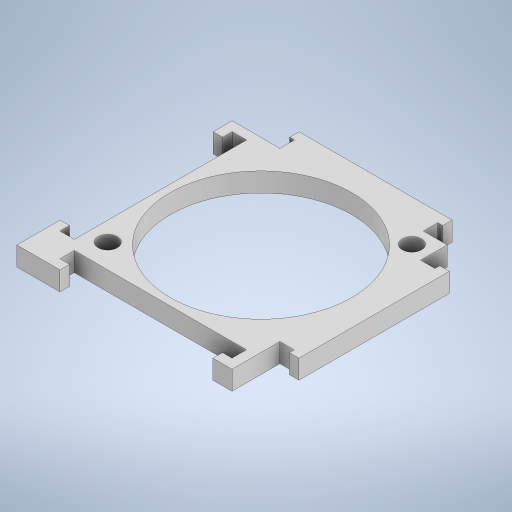
# Autodesk Inventor part: Maschio-femmina
Saved by Autodesk Inventor 2024 (Build 280153000, 153)
## iProperties
Created: 2024-01-14
Part Number: Maschio-femmina
Material: Generico
Document SubType Name: Modeling
Designer: Leonardo
Density: 1 g/cm^3
Appearance: Default
Author: Leonardo
Autodesk Inventor part; units mm, degrees
ref_plane "YZ Plane" through (0, 0, 0) normal (1, 0, 0) x (0, 1, 0)
ref_plane "XZ Plane" through (0, 0, 0) normal (0, 1, 0) x (-1, 0, 0)
ref_plane "XY Plane" through (0, 0, 0) normal (0, 0, 1) x (1, 0, 0)
sketch "Schizzo1" plane through (0, 0, 0) normal (0, 1, 0) x (-1, 0, 0)
  line L0 (10.0009, -10.0148) -> (9.0009, -10.0148)
  line L1 (-10, 9) -> (-10, 10)
  line L2 (11.5009, -9.0148) -> (10.0009, -9.0148)
  line L3 (10.0009, 8.9852) -> (10.0009, -9.0148)
  line L4 (-10, 12) -> (-10, 10)
  line L5 (9, 10) -> (-9, 10)
  line L6 (-10, -10.0148) -> (-9, -10.0148)
  line L7 (9.0009, -10.0148) -> (8.0009, -10.0148)
  line L8 (-9, -10.0148) -> (-8, -10.0148)
  line L9 (-10, 9) -> (-10, 8)
  line L10 (-10, -10.0148) -> (-10, -7.7324)
  circle A0 centre (-0.2724, -0.2591) radius 9.5
  line L11 (11.5009, -9.0148) -> (11.5009, -8.0148)
  line L12 (11.5009, -8.0148) -> (12.5009, -8.0148)
  line L13 (12.5009, -8.0148) -> (12.5009, -10.0148)
  line L14 (12.5009, -10.0148) -> (10.0009, -10.0148)
  line L15 (10.0009, 8.9852) -> (11.5009, 8.9852)
  line L16 (11.5009, 8.9852) -> (11.5009, 7.9852)
  line L17 (11.5009, 7.9852) -> (12.5009, 7.9852)
  line L18 (12.5009, 7.9852) -> (12.5009, 9.9852)
  line L19 (9, 10) -> (9, 11.5)
  line L20 (9, 11.5) -> (8, 11.5)
  line L21 (8, 11.5) -> (8, 12.5)
  line L22 (8, 12.5) -> (10, 12.5)
  line L23 (12.5009, 9.9852) -> (12.5009, 12.5)
  line L24 (12.5009, 12.5) -> (10, 12.5)
  line L25 (-9, 10) -> (-9, 11.5)
  line L26 (-9, 11.5) -> (-8, 11.5)
  line L27 (-8, 11.5) -> (-8, 12.5)
  line L28 (-8, 12.5) -> (-10, 12.5)
  line L29 (-10, 12.5) -> (-10, 12)
  line L30 (-10, -7.7324) -> (-10, -7.2324)
  line L31 (-10, 8) -> (-10, 7.5)
  line L32 (-10, 7.5) -> (-11, 7.5)
  line L33 (8.0009, -10.0148) -> (7.5009, -10.0148)
  line L34 (7.5009, -10.0148) -> (7.5009, -11.0148)
  line L35 (-8, -10.0148) -> (-7.5, -10.0148)
  line L36 (-7.5, -10.0148) -> (-7.5, -11.0148)
  line L37 (-10, -7.2324) -> (-11.5, -7.2324)
  line L38 (-11.5, -7.2324) -> (-11.5, -7.7324)
  line L39 (-11.5, -7.7324) -> (-12.5, -7.7324)
  line L40 (-11, 7.5) -> (-11.5, 7.5)
  line L41 (-11.5, 7.5) -> (-11.5, 8)
  line L42 (-11.5, 8) -> (-12.5, 8)
  line L43 (-12.5, -7.7324) -> (-12.5, 8)
  line L44 (-7.5, -11.0148) -> (-7.5, -11.5148)
  line L45 (-7.5, -11.5148) -> (-8, -11.5148)
  line L46 (-8, -11.5148) -> (-8, -12.5148)
  line L47 (7.5009, -11.0148) -> (7.5009, -11.5148)
  line L48 (7.5009, -11.5148) -> (8.0009, -11.5148)
  line L49 (8.0009, -11.5148) -> (8.0009, -12.5148)
  line L50 (8.0009, -12.5148) -> (-8, -12.5148)
  circle A1 centre (-8.1016, -8.2148) radius 1
  circle A2 centre (8.0009, 7.5) radius 1
  point P0 (0, 0)
  dimension "d24" = 1.5
  dimension "d36" = 1
  dimension "d43" = 1
  dimension "d44" = 1
  dimension "d45" = 2
  dimension "d46" = 1
  dimension "d47" = 1.5
  dimension "d48" = 1
  dimension "d49" = 1
  dimension "d51" = 1.5
  dimension "d53" = 1
  dimension "d54" = 2
  dimension "d55" = 0.5
  dimension "d56" = 0.5
  dimension "d59" = 0.5
  dimension "d65" = 1.5
  dimension "d66" = 0.5
  dimension "d67" = 0.5
  dimension "d70" = 0.5
  dimension "d71" = 0.5
  dimension "d72" = 2
  dimension "d73" = 2
  constraints: 102 end point, 17 perpendicular, 12 horizontal, 11 vertical, 3 centre point
  measures "d24" distance of L2.start L2.end
  measures "d36" distance of L0.end L7.end
  measures "d43" distance of L2.start L11.end
  measures "d44" distance of L11.end L12.end
  measures "d45" distance of L12.end L13.end
  measures "d46" distance of L15.end L16.end
  measures "d47" distance of L5.start L19.end
  measures "d48" distance of L19.end L20.end
  measures "d49" distance of L20.end L21.end
  measures "d51" distance of L5.end L25.end
  measures "d53" distance of L25.end L26.end
  measures "d54" distance of L27.end L28.end
  measures "d55" distance of L10.end L30.end
  measures "d56" distance of L9.end L31.end
  measures "d59" distance of L8.end L35.end
  measures "d65" distance of L30.end L37.end
  measures "d66" distance of L32.end L40.end
  measures "d67" distance of L40.end L41.end
  measures "d70" distance of L36.end L44.end
  measures "d71" distance of L44.end L45.end
  measures "d72" diameter of A1
  measures "d73" diameter of A2
extrude "Estrusione5" add sketch "Schizzo1" along normal blind 2
